Autodesk Fusion 360 part; units mm, degrees
note: some values were not read from the file. Set by a fixed rule: which face or edge a step refers to.
(part 2 of 2)
sketch "Skizze30" plane through (0, 0, 6.5) normal (0, 0, 1) x (-1, 0, 0)
  arc A0 (-2, -91.05) -> (5.05, -84) centre (-2, -84) ccw
  line L0 (-2, -91.05) -> (-48, -91.05)
  arc A1 (-55.05, -84) -> (-48, -91.05) centre (-48, -84) ccw
  line L1 (-55.05, -84) -> (-55.05, -2)
  arc A2 (-48, 5.05) -> (-55.05, -2) centre (-48, -2) ccw
  line L2 (-48, 5.05) -> (-2, 5.05)
  arc A3 (5.05, -2) -> (-2, 5.05) centre (-2, -2) ccw
  line L3 (5.05, -2) -> (5.05, -84)
  arc A4 (15.25, 1.0661) -> (10.25, 6.0661) centre (10.25, 1.0661) ccw
  line L4 (10.25, 6.0661) -> (-60.25, 6.0661)
  arc A5 (-60.25, 6.0661) -> (-65.25, 1.0661) centre (-60.25, 1.0661) ccw
  line L5 (-65.25, 1.0661) -> (-65.25, -87.0661)
  arc A6 (-65.25, -87.0661) -> (-60.25, -92.0661) centre (-60.25, -87.0661) ccw
  line L6 (-60.25, -92.0661) -> (10.25, -92.0661)
  arc A7 (10.25, -92.0661) -> (15.25, -87.0661) centre (10.25, -87.0661) ccw
  line L7 (15.25, -87.0661) -> (15.25, 1.0661)
  arc A8 (-2, -90.05) -> (4.05, -84) centre (-2, -84) ccw
  line L8 (-2, -90.05) -> (-48, -90.05)
  arc A9 (-54.05, -84) -> (-48, -90.05) centre (-48, -84) ccw
  line L9 (-54.05, -84) -> (-54.05, -2)
  arc A10 (-48, 4.05) -> (-54.05, -2) centre (-48, -2) ccw
  line L10 (-48, 4.05) -> (-2, 4.05)
  arc A11 (4.05, -2) -> (-2, 4.05) centre (-2, -2) ccw
  line L11 (4.05, -2) -> (4.05, -84)
  line L12 (5.05, -84) -> (5.05, -2)
  arc A12 (5.05, -2) -> (-2, 5.05) centre (-2, -2) ccw
  line L13 (-2, 5.05) -> (-48, 5.05)
  arc A13 (-48, 5.05) -> (-55.05, -2) centre (-48, -2) ccw
  line L14 (-55.05, -2) -> (-55.05, -84)
  arc A14 (-55.05, -84) -> (-48, -91.05) centre (-48, -84) ccw
  line L15 (-48, -91.05) -> (-2, -91.05)
  arc A15 (-2, -91.05) -> (5.05, -84) centre (-2, -84) ccw
  line L16 (-56.05, -84) -> (-56.05, -2)
  arc A16 (-48, 6.05) -> (-56.05, -2) centre (-48, -2) ccw
  line L17 (-48, 6.05) -> (-2, 6.05)
  arc A17 (6.05, -2) -> (-2, 6.05) centre (-2, -2) ccw
  line L18 (6.05, -2) -> (6.05, -84)
  arc A18 (-2, -92.05) -> (6.05, -84) centre (-2, -84) ccw
  line L19 (-2, -92.05) -> (-48, -92.05)
  arc A19 (-56.05, -84) -> (-48, -92.05) centre (-48, -84) ccw
  arc A20 (-48, 7.05) -> (-57.05, -2) centre (-48, -2) ccw
  line L20 (-57.05, -84) -> (-57.05, -2)
  arc A21 (-57.05, -84) -> (-48, -93.05) centre (-48, -84) ccw
  line L21 (-2, -93.05) -> (-48, -93.05)
  arc A22 (-2, -93.05) -> (7.05, -84) centre (-2, -84) ccw
  line L22 (7.05, -2) -> (7.05, -84)
  arc A23 (7.05, -2) -> (-2, 7.05) centre (-2, -2) ccw
  line L23 (-48, 7.05) -> (-2, 7.05)
  arc A24 (-48, 8.05) -> (-58.05, -2) centre (-48, -2) ccw
  line L24 (-58.05, -84) -> (-58.05, -2)
  arc A25 (-58.05, -84) -> (-48, -94.05) centre (-48, -84) ccw
  line L25 (-2, -94.05) -> (-48, -94.05)
  arc A26 (-2, -94.05) -> (8.05, -84) centre (-2, -84) ccw
  line L26 (8.05, -2) -> (8.05, -84)
  arc A27 (8.05, -2) -> (-2, 8.05) centre (-2, -2) ccw
  line L27 (-48, 8.05) -> (-2, 8.05)
  arc A28 (-48, 9.05) -> (-59.05, -2) centre (-48, -2) ccw
  line L28 (-59.05, -84) -> (-59.05, -2)
  arc A29 (-59.05, -84) -> (-48, -95.05) centre (-48, -84) ccw
  line L29 (-2, -95.05) -> (-48, -95.05)
  arc A30 (-2, -95.05) -> (9.05, -84) centre (-2, -84) ccw
  line L30 (9.05, -2) -> (9.05, -84)
  arc A31 (9.05, -2) -> (-2, 9.05) centre (-2, -2) ccw
  line L31 (-48, 9.05) -> (-2, 9.05)
  arc A32 (-48, 10.05) -> (-60.05, -2) centre (-48, -2) ccw
  line L32 (-60.05, -84) -> (-60.05, -2)
  arc A33 (-60.05, -84) -> (-48, -96.05) centre (-48, -84) ccw
  line L33 (-2, -96.05) -> (-48, -96.05)
  arc A34 (-2, -96.05) -> (10.05, -84) centre (-2, -84) ccw
  line L34 (10.05, -2) -> (10.05, -84)
  arc A35 (10.05, -2) -> (-2, 10.05) centre (-2, -2) ccw
  line L35 (-48, 10.05) -> (-2, 10.05)
  arc A36 (-48, 11.05) -> (-61.05, -2) centre (-48, -2) ccw
  line L36 (-61.05, -84) -> (-61.05, -2)
  arc A37 (-61.05, -84) -> (-48, -97.05) centre (-48, -84) ccw
  line L37 (-2, -97.05) -> (-48, -97.05)
  arc A38 (-2, -97.05) -> (11.05, -84) centre (-2, -84) ccw
  line L38 (11.05, -2) -> (11.05, -84)
  arc A39 (11.05, -2) -> (-2, 11.05) centre (-2, -2) ccw
  line L39 (-48, 11.05) -> (-2, 11.05)
  arc A40 (-48, 12.05) -> (-62.05, -2) centre (-48, -2) ccw
  line L40 (-62.05, -84) -> (-62.05, -2)
  arc A41 (-62.05, -84) -> (-48, -98.05) centre (-48, -84) ccw
  line L41 (-2, -98.05) -> (-48, -98.05)
  arc A42 (-2, -98.05) -> (12.05, -84) centre (-2, -84) ccw
  line L42 (12.05, -2) -> (12.05, -84)
  arc A43 (12.05, -2) -> (-2, 12.05) centre (-2, -2) ccw
  line L43 (-48, 12.05) -> (-2, 12.05)
  arc A44 (-48, 13.05) -> (-63.05, -2) centre (-48, -2) ccw
  line L44 (-63.05, -84) -> (-63.05, -2)
  arc A45 (-63.05, -84) -> (-48, -99.05) centre (-48, -84) ccw
  line L45 (-2, -99.05) -> (-48, -99.05)
  arc A46 (-2, -99.05) -> (13.05, -84) centre (-2, -84) ccw
  line L46 (13.05, -2) -> (13.05, -84)
  arc A47 (13.05, -2) -> (-2, 13.05) centre (-2, -2) ccw
  line L47 (-48, 13.05) -> (-2, 13.05)
  arc A48 (-48, 14.05) -> (-64.05, -2) centre (-48, -2) ccw
  line L48 (-64.05, -84) -> (-64.05, -2)
  arc A49 (-64.05, -84) -> (-48, -100.05) centre (-48, -84) ccw
  line L49 (-2, -100.05) -> (-48, -100.05)
  arc A50 (-2, -100.05) -> (14.05, -84) centre (-2, -84) ccw
  line L50 (14.05, -2) -> (14.05, -84)
  arc A51 (14.05, -2) -> (-2, 14.05) centre (-2, -2) ccw
  line L51 (-48, 14.05) -> (-2, 14.05)
  line L52 (-65.25, -87.0661) -> (-65.25, 1.0661)
  arc A52 (-60.25, 6.0661) -> (-65.25, 1.0661) centre (-60.25, 1.0661) ccw
  line L53 (-60.25, 6.0661) -> (10.25, 6.0661)
  arc A53 (15.25, 1.0661) -> (10.25, 6.0661) centre (10.25, 1.0661) ccw
  line L54 (15.25, 1.0661) -> (15.25, -87.0661)
  arc A54 (10.25, -92.0661) -> (15.25, -87.0661) centre (10.25, -87.0661) ccw
  line L55 (10.25, -92.0661) -> (-60.25, -92.0661)
  arc A55 (-65.25, -87.0661) -> (-60.25, -92.0661) centre (-60.25, -87.0661) ccw
  line L56 (-60.25, -91.0661) -> (10.25, -91.0661)
  arc A56 (10.25, -91.0661) -> (14.25, -87.0661) centre (10.25, -87.0661) ccw
  line L57 (14.25, -87.0661) -> (14.25, 1.0661)
  arc A57 (14.25, 1.0661) -> (10.25, 5.0661) centre (10.25, 1.0661) ccw
  line L58 (10.25, 5.0661) -> (-60.25, 5.0661)
  arc A58 (-60.25, 5.0661) -> (-64.25, 1.0661) centre (-60.25, 1.0661) ccw
  line L59 (-64.25, 1.0661) -> (-64.25, -87.0661)
  arc A59 (-64.25, -87.0661) -> (-60.25, -91.0661) centre (-60.25, -87.0661) ccw
  dimension "d252" = 1
  dimension "d253" = -2
  dimension "d254" = -3
  dimension "d255" = -4
  dimension "d256" = -5
  dimension "d257" = -6
  dimension "d258" = -7
  dimension "d259" = -8
  dimension "d260" = -9
  dimension "d261" = -1
extrude "Extrusion12'" add sketch "Skizze30" along normal blind 4 contours A4 A7 L7 A50 A51 A53 L54 A54 A56 L57 A57 | A4 A47 A51 A53 A57 | A4 L4 A43 A47 L53 A53 A57 L58 | A50 L50 A51 A56 L57 A57 | A7 A46 A50 A54 A56 | A42 L42 A43 A46 L46 A47 L56 A56 A57 L58 | L6 A7 A42 A46 A54 L55 L56 A56 | L4 A39 A43 L53 L58 | A5 L5 A6 A48 A49 L52 A52 A55 A58 L59 A59 | A5 A44 A48 A52 A58 | L4 A35 A39 L53 L58 | L4 A5 A40 A44 A52 L53 L58 A58 | A48 L48 A49 A58 L59 A59 | L6 A38 A42 L55 L56 | A6 A45 A49 A55 A59 | L4 A31 A35 L53 L58 | A34 L34 A35 A38 L38 A39 L56 L58 | A40 L40 A41 A44 L44 A45 L56 L58 A58 A59 | L6 A34 A38 L55 L56 | A6 L6 A41 A45 L55 A55 L56 A59 | L4 A27 A31 L53 L58 | L4 A36 A40 L53 L58 | L6 A30 A34 L55 L56 | L4 A23 A27 L53 L58 | A26 L26 A27 A30 L30 A31 L56 L58 | L4 A32 A36 L53 L58 | L6 A26 A30 L55 L56 | L6 A37 A41 L55 L56 | L4 A16 L17 A17 A20 A23 L53 L58 | L4 A28 A32 L53 L58 | A32 L32 A33 A36 L36 A37 L56 L58 | L6 A22 A26 L55 L56 | L6 A33 A37 L55 L56 | L4 A20 A24 L53 L58 | A17 L18 A18 A22 L22 A23 L56 L58 | L4 A24 A28 L53 L58 | L6 A18 L19 A19 A21 A22 L55 L56 | L6 A29 A33 L55 L56 | L16 A16 A19 A20 L20 A21 L56 L58 | A16 L17 A17 L58 | A24 L24 A25 A28 L28 A29 L56 L58 | L6 A21 A25 L55 L56 | L6 A25 A29 L55 L56 | A18 L19 A19 L56 bodies 4 in component "Outer Body"
component "Case" placed x (1, 0, 0) y (0, 1, 0) z (0, 0, 1) at (0, 0, 0)
component "Inner Body" placed x (1, 0, 0) y (0, 1, 0) z (0, 0, 1) at (0, 0, 0) in component "Case"
component "Outer Body" placed x (1, 0, 0) y (0, 1, 0) z (0, 0, 1) at (0, 0, 0) in component "Case"
named bodies: "Inner Body", "Outer Body"
